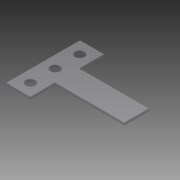
# Autodesk Inventor part: pto finger
Saved by Autodesk Inventor 2014 SP1 (Build 180222100, 222)
## iProperties
Created: 2014-03-10
Part Number: pto finger
Material: Generic
Document SubType Name: Modeling
Designer: Ryan
Density: 1 g/cm^3
Appearance: Polycarbonate - Clear
Author: Ryan
Autodesk Inventor part; units mm, degrees
ref_plane "YZ Plane" through (0, 0, 0) normal (1, 0, 0) x (0, 1, 0)
ref_plane "XZ Plane" through (0, 0, 0) normal (0, 1, 0) x (-1, 0, 0)
ref_plane "XY Plane" through (0, 0, 0) normal (0, 0, 1) x (1, 0, 0)
sketch "Sketch1" plane through (0, 0, 0) normal (0, 1, 0) x (-1, 0, 0)
  line L0 (-16.2942, -22.7333) -> (-28.9942, -22.7333)
  line L1 (-28.9942, 2.6667) -> (-16.2942, 2.6667)
  line L2 (-16.2942, 2.6667) -> (-16.2942, -22.7333)
  line L3 (-16.2942, -22.7333) -> (-28.9942, 2.6667) construction
  line L4 (-28.9942, -22.7333) -> (-16.2942, 2.6667) construction
  line L5 (-79.7942, -15.1133) -> (-79.7942, 2.6667)
  line L6 (-79.7942, -15.1133) -> (-28.9942, -15.1133)
  line L7 (-79.7942, 2.6667) -> (-28.9942, 2.6667)
  line L8 (-28.9942, -22.7333) -> (-28.9942, -15.1133)
  line L9 (-28.9942, 2.6667) -> (-28.9942, 2.6667)
  line L10 (-28.9942, 2.6667) -> (-16.2942, 2.6667)
  line L11 (-16.2942, 2.6667) -> (-16.2942, 15.3667)
  line L12 (-16.2942, 15.3667) -> (-28.9942, 15.3667)
  line L13 (-28.9942, 15.3667) -> (-28.9942, 2.6667)
  point P0 (-22.6442, -10.0333)
  dimension "d2" = 12.7
  dimension "d4" = 17.78
  dimension "d6" = 50.8
  dimension "d7" = 26.565
  dimension "d19" = 12.7
  constraints: 28 end point, 6 parallel, 5 perpendicular, 3 collinear, 2 horizontal, 2 midpoint
  measures "d2" distance of L1.start L1.end
  measures "d4" distance of L5.start L5.end
  measures "d6" distance between parallel lines of L9 L5
  measures "d7" angle of L3 L2
  measures "d19" distance between parallel lines of L12 L7
extrude "Extrusion1" add sketch "Sketch1" along normal blind 1.5875
sketch "Sketch2" plane through (0, 1.5875, 0) normal (0, 1, 0) x (1, 0, 0)
  line L0 (28.9942, -2.6667) -> (16.2942, -2.6667)
  line L1 (16.2942, -2.6667) -> (16.2942, 22.7333)
  line L2 (16.2942, 22.7333) -> (28.9942, 22.7333)
  line L3 (28.9942, 22.7333) -> (28.9942, -2.6667)
  line L4 (28.9942, -2.6667) -> (16.2942, 22.7333) construction
  line L5 (16.2942, -2.6667) -> (28.9942, 22.7333) construction
  line L6 (22.6442, -2.6667) -> (22.6442, 22.7333) construction
  circle A0 centre (22.6442, 16.3833) radius 2.3114
  circle A1 centre (22.6442, 3.6833) radius 2.3114
  circle A2 centre (22.6442, -9.0167) radius 2.3114
  point P0 (16.2942, -2.6667)
  point P1 (0, 0)
  point P2 (22.6442, 10.0333)
  dimension "d11" = 6.35
  dimension "d12" = 4.6228
  dimension "d22" = 12.7
  constraints: 14 end point, 4 midpoint, 3 centre point, 2 parallel, 1 horizontal, 1 perpendicular, 1 point on line, 1 vertical, 4 other
  measures "d11" distance between parallel lines of L1 L6
  measures "d12" diameter of A0
  measures "d22" distance of A0.centre A1.centre
extrude "Extrusion2" cut sketch "Sketch2" against normal blind 1.5875 contours A0 | A1 | A2
sketch "Sketch3" plane through (0, 0, 0) normal (0, -1, 0) x (1, 0, 0)
  line L0 (79.7942, -15.1133) -> (28.9942, -15.1133) projected
  line L1 (79.7942, 2.6667) -> (79.7942, -15.1133) projected
  line L2 (28.9942, -15.1133) -> (79.7942, -15.1133)
  line L3 (79.7942, -15.1133) -> (79.7942, -10.0333)
  line L4 (79.7942, -10.0333) -> (28.9942, -10.0333)
  line L5 (28.9942, -10.0333) -> (28.9942, -15.1133)
  point P0 (0, 0)
  dimension "d27" = 5.08
  constraints: 8 end point, 2 parallel, 1 horizontal, 1 perpendicular, 1 point on line
  measures "d27" distance of L4.end L0.end
extrude "Extrusion3" cut sketch "Sketch3" against normal blind 1.5875
sketch "Sketch4" plane through (0, 0, 0) normal (0, -1, 0) x (1, 0, 0)
  line L0 (83.7791, 7.7007) -> (64.7085, 7.7007)
  line L1 (64.7085, 7.7007) -> (64.7085, -14.0719)
  line L2 (64.7085, -14.0719) -> (83.7791, -14.0719)
  line L3 (83.7791, -14.0719) -> (83.7791, 7.7007)
  point P0 (0, 0)
  constraints: 8 end point, 2 parallel, 1 horizontal, 1 perpendicular
extrude "Extrusion4" cut sketch "Sketch4" against normal blind 1.5875
fillet "Fillet2" radius 0.381 30 edges at (64.7085, 0, -3.6833) (46.8514, 0, 2.6667) (28.9942, 0, 9.0167) (22.6442, 0, 15.3667) (16.2942, 0, -3.6833) (22.6442, 0, -22.7333) (28.9942, 0, -16.3833) (46.8514, 0, -10.0333) (64.7085, 0.7937, 2.6667) (46.8514, 1.5875, 2.6667) (28.9942, 0.7937, 2.6667) (64.7085, 1.5875, -3.6833) (46.8514, 1.5875, -10.0333) (28.9942, 1.5875, -16.3833) (22.6442, 1.5875, -22.7333) (16.2942, 1.5875, -3.6833) (22.6442, 1.5875, 15.3667) (28.9942, 1.5875, 9.0167) (64.7085, 0.7937, -10.0333) (28.9942, 0.7937, -10.0333) (20.3328, 1.5875, -16.3833) (20.3328, 0, -16.3833) (16.2942, 0.7937, -22.7333) (28.9942, 0.7937, -22.7333) (16.2942, 0.7937, 15.3667) (20.3328, 1.5875, -3.6833) (20.3328, 0, -3.6833) (20.3328, 1.5875, 9.0167) (20.3328, 0, 9.0167) (28.9942, 0.7937, 15.3667)
body "Solid1"
